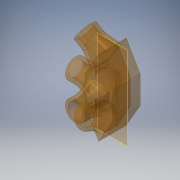
# Autodesk Inventor part: ThreePipeAdapter2
Saved by Autodesk Inventor 2016 (Build 200138000, 138)
## iProperties
Created: 2017-10-02
Part Number: ThreePipeAdapter2
Material: Polycarbonate, Smoke
Document SubType Name: Modeling
Designer: reinert
Density: 1.2 g/cm^3
Appearance: Polycarbonate - Smoked
Author: reinert
Autodesk Inventor part; units mm, degrees
ref_plane "YZ Plane" through (0, 0, 0) normal (1, 0, 0) x (0, 1, 0)
ref_plane "XZ Plane" through (0, 0, 0) normal (0, 1, 0) x (-1, 0, 0)
ref_plane "XY Plane" through (0, 0, 0) normal (0, 0, 1) x (1, 0, 0)
sketch "Sketch1" plane through (0, 0, 0) normal (0, 1, 0) x (-1, 0, 0)
  line L0 (7.940122, -4.573632) -> (37.940122, -4.573632)
  line L1 (37.940122, -4.573632) -> (37.940122, -34.573632)
  line L2 (37.940122, -34.573632) -> (7.940122, -34.573632)
  line L3 (7.940122, -34.573632) -> (7.940122, -4.573632)
  line L4 (37.940122, -4.573632) -> (22.940122, 21.40713)
  line L5 (37.940122, -4.573632) -> (67.940122, -4.573632) construction
  line L6 (22.940122, 21.40713) -> (7.940122, -4.573632)
  line L7 (37.940122, -34.573632) -> (22.940122, -60.554394)
  line L8 (37.940122, -34.573632) -> (67.940122, -34.573632) construction
  line L9 (22.940122, -60.554394) -> (7.940122, -34.573632)
  dimension "d6" = 30
  dimension "d7" = 30
  dimension "d8" = 30
  dimension "d9" = 120
  dimension "d10" = 30
  dimension "d11" = 120
  constraints: 20 end point, 3 horizontal, 3 parallel, 2 equal length, 1 perpendicular
  measures "d6" distance of L1.end L2.end
  measures "d7" distance of L0.end L1.end
  measures "d8" distance of L0.end L4.end
  measures "d9" angle of L5 L4
  measures "d10" distance of L1.end L7.end
  measures "d11" angle of L7 L8
sketch "Sketch1 outline for Extrusion1" plane through (0, 0, 0) normal (0, 1, 0) x (-1, 0, 0)
  line L0 (22.940122, 21.40713) -> (7.940122, -4.573632)
  line L1 (7.940122, -4.573632) -> (7.940122, -34.573632)
  line L2 (7.940122, -34.573632) -> (22.940122, -60.554394)
  line L3 (22.940122, -60.554394) -> (37.940122, -34.573632)
  line L4 (37.940122, -34.573632) -> (37.940122, -4.573632)
  line L5 (37.940122, -4.573632) -> (22.940122, 21.40713)
extrude "Extrusion1" add sketch "Sketch1 outline for Extrusion1" along normal blind 30
sketch "Sketch2" plane through (-37.940122, 0, -34.573632) normal (-1, 0, 0) x (0, 0, 1)
  circle A0 centre (15, 15) radius 15
  line L0 (0, 30) -> (-25.980762, 30)
  line L1 (30, 0) -> (55.980762, 0)
  line L2 (0, 30) -> (30, 0)
  line L3 (0, 0) -> (-25.980762, 0)
  line L4 (30, 30) -> (55.980762, 30)
  line L5 (0, 0) -> (30, 30)
  point P0 (34.573632, 0)
  dimension "d15" = 30
  constraints: 4 end point, 1 centre point, 1 midpoint
  measures "d15" diameter of A0
sketch "Sketch2 outline for Extrusion2" plane through (-37.940122, 0, -34.573632) normal (-1, 0, 0) x (0, 0, 1)
  circle A0 centre (15, 15) radius 15
extrude "Extrusion2" add sketch "Sketch2 outline for Extrusion2" along normal blind 15 draft -15
sketch "Sketch4" plane through (-52.940122, 15, -19.573632) normal (-1, 0, 0) x (0, 0, 1)
  circle A0 centre (0, 0) radius 7.874934
  circle A1 centre (0, 0) radius 10.980762
  point P0 (19.573632, -15)
  constraints: 2 centre point, 1 coincident
sketch "Sketch4 outline for Extrusion4" plane through (-52.940122, 15, -19.573632) normal (-1, 0, 0) x (0, 0, 1)
  circle A0 centre (0, 0) radius 10.980762
  circle A1 centre (0, 0) radius 7.874934
extrude "Extrusion4" add sketch "Sketch4 outline for Extrusion4" along normal blind 10
sketch "Sketch6" plane through (0, 0, 0) normal (0, -1, 0) x (1, 0, 0)
  line L0 (-7.940122, -34.573632) -> (-22.940122, -60.554394)
  line L1 (-7.940122, -34.573632) -> (-37.806391, -4.849081)
  line L2 (-37.940122, -34.573632) -> (-37.940122, -19.573632)
  line L3 (-37.940122, -34.573632) -> (-8.205449, -4.849081)
  circle A0 centre (-23.072786, -19.711356) radius 15
  point P0 (0, 0)
  dimension "d26" = 30
  constraints: 4 end point, 1 centre point, 1 midpoint
  measures "d26" diameter of A0
sketch "Sketch6 outline for Extrusion5" plane through (0, 0, 0) normal (0, -1, 0) x (1, 0, 0)
  circle A0 centre (-23.072786, -19.711356) radius 15
extrude "Extrusion5" add sketch "Sketch6 outline for Extrusion5" along normal blind 15 draft -15
sketch "Sketch7" plane through (-22.940122, 0, -60.554394) normal (-0.8660254, 0, -0.5) x (-0.5, 0, 0.8660254)
  line L0 (0, 30) -> (30, 30) projected
  line L1 (15, 0) -> (0, 0) projected
  line L2 (30, 30) -> (0, 0)
  line L3 (15, 30) -> (0, 30) projected
  line L4 (0, 0) -> (30, 0) projected
  line L5 (0, 30) -> (30, 0)
  line L6 (15, 0) -> (15, 30) projected
  circle A0 centre (15, 15) radius 15
  point P0 (40.971583, 0)
  dimension "d29" = 30
  constraints: 4 end point, 1 centre point, 1 midpoint
  measures "d29" diameter of A0
sketch "Sketch7 outline for Extrusion6" plane through (-22.940122, 0, -60.554394) normal (-0.8660254, 0, -0.5) x (-0.5, 0, 0.8660254)
  circle A0 centre (15, 15) radius 15
extrude "Extrusion6" add sketch "Sketch7 outline for Extrusion6" along normal blind 15 draft -15
sketch "Sketch8" plane through (-22.940122, 0, 21.40713) normal (-0.8660254, 0, 0.5) x (0.5, 0, 0.8660254)
  line L0 (-42.990381, 30) -> (-30, 30)
  line L1 (0, 0) -> (0, 30)
  line L2 (-30, 30) -> (0, 0)
  line L3 (-30.081643, 0) -> (0, 30)
  circle A0 centre (-15.040821, 15) radius 15
  point P0 (-7.069057, 0)
  dimension "d32" = 30
  constraints: 4 end point, 1 centre point, 1 midpoint
  measures "d32" diameter of A0
sketch "Sketch8 outline for Extrusion7" plane through (-22.940122, 0, 21.40713) normal (-0.8660254, 0, 0.5) x (0.5, 0, 0.8660254)
  circle A0 centre (-15.040821, 15) radius 15
extrude "Extrusion7" add sketch "Sketch8 outline for Extrusion7" along normal blind 15 draft -15
sketch "Sketch9" plane through (-52.940122, 15, -19.573632) normal (-1, 0, 0) x (0, 0, 1)
  circle A0 centre (0, 0) radius 7.874934
  point P0 (19.573632, -15)
  constraints: 1 centre point
sketch "Sketch9 outline for Extrusion8" plane through (-52.940122, 15, -19.573632) normal (-1, 0, 0) x (0, 0, 1)
  circle A0 centre (0, 0) radius 7.874934
extrude "Extrusion8" cut sketch "Sketch9 outline for Extrusion8" against normal blind 25 draft 15
sketch "Sketch10" plane through (-43.430503, 15, -55.064013) normal (-0.8660254, 0, -0.5) x (-0.5, 0, 0.8660254)
  circle A0 centre (0, 0) radius 7.875
  circle A1 centre (0, 0) radius 10.980762
  point P0 (25.971583, -15)
  dimension "d37" = 15.75
  constraints: 2 centre point, 1 coincident
  measures "d37" diameter of A0
sketch "Sketch10 outline for Extrusion9" plane through (-43.430503, 15, -55.064013) normal (-0.8660254, 0, -0.5) x (-0.5, 0, 0.8660254)
  circle A0 centre (0, 0) radius 10.980762
  circle A1 centre (0, 0) radius 7.875
extrude "Extrusion9" add sketch "Sketch10 outline for Extrusion9" along normal blind 10
sketch "Sketch11" plane through (-43.430503, 15, -55.064013) normal (-0.8660254, 0, -0.5) x (-0.5, 0, 0.8660254)
  line L0 (0, -15) -> (0, 15) projected
  circle A0 centre (0, 0) radius 7.875
  point P0 (25.971583, -15)
  constraints: 1 centre point, 1 midpoint
sketch "Sketch11 outline for Extrusion10" plane through (-43.430503, 15, -55.064013) normal (-0.8660254, 0, -0.5) x (-0.5, 0, 0.8660254)
  circle A0 centre (0, 0) radius 7.875
extrude "Extrusion10" cut sketch "Sketch11 outline for Extrusion10" against normal blind 15 draft 15
ref_plane "Work Plane1" through (0, 15, 0) normal (0, -1, 0) x (1, 0, 0)
sketch "Sketch12" plane through (0, 15, 0) normal (0, -1, 0) x (1, 0, 0)
  line L0 (-52.940122, -11.698699) -> (-27.940122, -4.999969)
  line L1 (-34.19829, -6.67684) -> (-34.190122, -41.068823)
  line L2 (-30.440122, -47.564013) -> (-37.940122, -34.573632)
  line L3 (-22.940122, -60.554394) -> (-30.440122, -47.564013)
  line L4 (-24.689014, -57.525226) -> (-11.004373, -33.083208)
  line L5 (-11.004373, -33.083208) -> (-11.011143, -4.573409)
  line L6 (-11.011143, -4.573409) -> (-24.689014, 18.377961)
  line L7 (-30.460533, 8.381396) -> (-22.940122, 21.40713)
  line L8 (-37.940122, -4.573632) -> (-30.460533, 8.381396)
  line L9 (-34.200328, 1.903882) -> (-34.19829, -6.67684)
  point P0 (0, 0)
  constraints: 10 end point, 3 point on line, 2 midpoint, 2 parallel
sketch "Sketch12 outline for Extrusion11" plane through (0, 15, 0) normal (0, -1, 0) x (1, 0, 0)
  line L0 (-34.200328, 1.903882) -> (-34.19829, -6.67684)
  line L1 (-30.460533, 8.381396) -> (-34.200328, 1.903882)
  line L2 (-24.689014, 18.377961) -> (-30.460533, 8.381396)
  line L3 (-11.011143, -4.573409) -> (-24.689014, 18.377961)
  line L4 (-11.004373, -33.083208) -> (-11.011143, -4.573409)
  line L5 (-24.689014, -57.525226) -> (-11.004373, -33.083208)
  line L6 (-30.440122, -47.564013) -> (-24.689014, -57.525226)
  line L7 (-34.190122, -41.068823) -> (-30.440122, -47.564013)
  line L8 (-34.19829, -6.67684) -> (-34.190122, -41.068823)
extrude "Extrusion11" cut sketch "Sketch12 outline for Extrusion11" along normal mid plane 15
sketch "Sketch13" plane through (-43.450914, 15, 15.881396) normal (-0.8660254, 0, 0.5) x (0.5, 0, 0.8660254)
  line L0 (0.040821, -15) -> (0.040821, 15)
  circle A0 centre (0.040821, 0) radius 11.021583
  circle A1 centre (0.040821, 0) radius 7.875
  point P0 (7.971764, -15)
  dimension "d45" = 15.75
  constraints: 2 centre point, 1 coincident, 1 midpoint
  measures "d45" diameter of A1
sketch "Sketch13 outline for Extrusion12" plane through (-43.450914, 15, 15.881396) normal (-0.8660254, 0, 0.5) x (0.5, 0, 0.8660254)
  circle A0 centre (0.040821, 0) radius 11.021583
  circle A1 centre (0.040821, 0) radius 7.875
extrude "Extrusion12" add sketch "Sketch13 outline for Extrusion12" along normal blind 10
sketch "Sketch14" plane through (-43.430503, 15, 15.916749) normal (-0.8660254, 0, 0.5) x (0.5, 0, 0.8660254)
  line L0 (0, -15) -> (0, 15) projected
  circle A0 centre (0, 0) radius 7.875
  point P0 (7.930943, -15)
  dimension "d48" = 15.75
  constraints: 1 centre point, 1 midpoint
  measures "d48" diameter of A0
sketch "Sketch14 outline for Extrusion13" plane through (-43.430503, 15, 15.916749) normal (-0.8660254, 0, 0.5) x (0.5, 0, 0.8660254)
  circle A0 centre (0, 0) radius 7.875
extrude "Extrusion13" cut sketch "Sketch14 outline for Extrusion13" against normal blind 15.75 draft 15
sketch "Sketch15" plane through (-23.072786, -15, -19.711356) normal (0, -1, 0) x (1, 0, 0)
  circle A0 centre (0, 0) radius 10.980762
  circle A1 centre (0, 0) radius 7.875
  point P0 (23.072786, 19.711356)
  dimension "d51" = 15.75
  constraints: 2 centre point, 1 coincident
  measures "d51" diameter of A1
sketch "Sketch15 outline for Extrusion14" plane through (-23.072786, -15, -19.711356) normal (0, -1, 0) x (1, 0, 0)
  circle A0 centre (0, 0) radius 10.980762
  circle A1 centre (0, 0) radius 7.875
extrude "Extrusion14" add sketch "Sketch15 outline for Extrusion14" along normal blind 10
sketch "Sketch16" plane through (-23.072786, -15, -19.711356) normal (0, -1, 0) x (1, 0, 0)
  circle A0 centre (0, 0) radius 7.875
  point P0 (23.072786, 19.711356)
  dimension "d54" = 15.75
  constraints: 1 centre point
  measures "d54" diameter of A0
sketch "Sketch16 outline for Extrusion15" plane through (-23.072786, -15, -19.711356) normal (0, -1, 0) x (1, 0, 0)
  circle A0 centre (0, 0) radius 7.875
extrude "Extrusion15" cut sketch "Sketch16 outline for Extrusion15" against normal blind 23 draft 15
equation "\"d49\" = d48"
body "Solid1"
